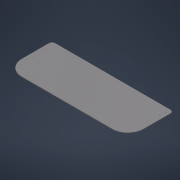
# Autodesk Inventor part: Base
Saved by Autodesk Inventor 2022 (Build 260153000, 153)
## iProperties
Created: 2021-09-08
Part Number: Base
Material: Steel, Mild, Welded
Document SubType Name: Modeling
Designer: Andres
Density: 7.85 g/cm^3
Appearance: Weld - Steel Mild
Author: Andres
Autodesk Inventor part; units mm, degrees
ref_plane "YZ Plane" through (0, 0, 0) normal (1, 0, 0) x (0, 1, 0)
ref_plane "XZ Plane" through (0, 0, 0) normal (0, 1, 0) x (-1, 0, 0)
ref_plane "XY Plane" through (0, 0, 0) normal (0, 0, 1) x (1, 0, 0)
sketch "Sketch1" plane through (0, 0, 0) normal (0, 1, 0) x (-1, 0, 0)
  line L0 (-380, -150) -> (380, -150)
  line L1 (400, -130) -> (400, 50)
  line L2 (300, 150) -> (-300, 150)
  line L3 (-400, 50) -> (-400, -130)
  line L4 (-400, -150) -> (400, 150) construction
  line L5 (400, -150) -> (-400, 150) construction
  arc A0 (400, 50) -> (300, 150) centre (300, 50) ccw
  arc A1 (-300, 150) -> (-400, 50) centre (-300, 50) ccw
  arc A2 (-400, -130) -> (-380, -150) centre (-380, -130) ccw
  arc A3 (380, -150) -> (400, -130) centre (380, -130) ccw
  line L6 (-300, 155) -> (300, 155)
  arc A4 (405, 50) -> (300, 155) centre (300, 50) ccw
  line L7 (405, 50) -> (405, -130)
  arc A5 (380, -155) -> (405, -130) centre (380, -130) ccw
  line L8 (380, -155) -> (-380, -155)
  arc A6 (-405, -130) -> (-380, -155) centre (-380, -130) ccw
  line L9 (-405, -130) -> (-405, 50)
  arc A7 (-300, 155) -> (-405, 50) centre (-300, 50) ccw
  point P0 (0, 0)
  point P1 (0, 0)
  dimension "d0" = 800
  dimension "d1" = 300
  dimension "d2" = 100
  dimension "d3" = 20
  dimension "espesor" = 5
  constraints: 20 end point, 16 point on circle, 8 centre point, 8 point on line, 8 tangent, 4 midpoint, 4 parallel, 2 equal radius, 2 perpendicular, 1 horizontal, 7 other
  measures "d0" distance of L4.end L5.end
  measures "d1" distance between parallel lines of L0 L2
  measures "d2" radius of A0
  measures "d3" radius of A2
  measures "espesor" distance between parallel lines of L1 L7
extrude "Extrusion1" add sketch "Sketch1" along normal blind 5 contours A2 L3 A1 L2 A0 L1 A3 L0
sketch "Sketch2" plane through (0, 5, 0) normal (0, 1, 0) x (1, 0, 0)
  line L0 (-290, -130) -> (-250, -130) construction
  line L1 (-300, -150) -> (300, -150) construction
  line L2 (0, 210) -> (0, -210) construction
  line L3 (290, -130) -> (250, -130) construction
  line L4 (-380, 120) -> (-380, 80) construction
  line L5 (-380, 0) -> (-380, -40) construction
  line L6 (-400, 130) -> (-400, -50) construction
  line L7 (380, 120) -> (380, 80) construction
  line L8 (380, 0) -> (380, -40) construction
  point P0 (0, 0)
  point P1 (-20, -130)
  point P2 (20, -130)
  dimension "d7" = 40
  dimension "d8" = 20
  dimension "d9" = 500
  dimension "d10" = 40
  dimension "d11" = 40
  dimension "d12" = 80
  dimension "d14" = 20
  dimension "d23" = 40
  constraints: 12 end point, 7 symmetric about line, 2 horizontal alignment, 2 vertical, 1 collinear, 1 horizontal
  measures "d7" distance of L0.start L0.end
  measures "d8" distance between parallel lines of L1 L0
  measures "d9" distance of L3.end L0.end
  measures "d10" distance of L5.start L5.end
  measures "d11" distance of L4.start L4.end
  measures "d12" distance of L5.start L4.end
  measures "d14" distance from line of L6 L5.end
  measures "d23" distance of point (20, -130) point (-20, -130)
hole "Hole1" at (-290, 5, 130) at (-250, 5, 130) at (290, 5, 130) at (250, 5, 130) at (-380, 5, -120) at (-380, 5, -80) at (-380, 5, 40) at (-380, 5, 0) at (380, 5, -120) at (380, 5, -80) at (380, 5, 0) at (380, 5, 40) at (-20, 5, 130) at (20, 5, 130) direction (0, -1, 0) diameter 3.4 end through all clearance for "Socket Head Cap Screw ISO 4762" size "M3" standard "ISO"
equation "\"d4\" = espesor"
equation "\"d10\" = d7"
equation "\"d11\" = d7"
equation "\"d23\" = d7"
body "Solid1"
